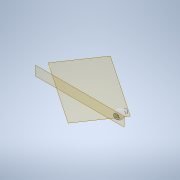
# Autodesk Inventor part: BallJoint
Saved by Autodesk Inventor 2020 (Build 240168000, 168)
## iProperties
Created: 2020-03-20
Part Number: BallJoint
Material: Generisch
Document SubType Name: Modeling
Designer: Fynn
Density: 1 g/cm^3
Appearance: Vorgabe
Author: Fynn
Autodesk Inventor part; units mm, degrees
ref_plane "YZ Plane" through (0, 0, 0) normal (1, 0, 0) x (0, 1, 0)
ref_plane "XZ Plane" through (0, 0, 0) normal (0, 1, 0) x (-1, 0, 0)
ref_plane "XY Plane" through (0, 0, 0) normal (0, 0, 1) x (1, 0, 0)
sketch "Skizze1" plane through (0, 0, 0) normal (0, 0, 1) x (1, 0, 0)
  circle A0 centre (75, -2.9684) radius 1.05 projected
  circle A1 centre (75, -2.9684) radius 2
  point P0 (0, 0)
  dimension "d0" = 4
  constraints: 1 centre point, 1 coincident
  measures "d0" diameter of A1
extrude "Extrusion1" add sketch "Skizze1" along normal blind 3
sketch "Skizze2" plane through (75, -2.9684, 3) normal (0, 0, 1) x (1, 0, 0)
  circle A0 centre (0, 0) radius 1.05 projected
  point P0 (-75, 2.9684)
ref_plane "Arbeitsebene2" through (75, -2.9684, 3) normal (-0.0001, 1, 0) x (-0.5613, -0.0001, 0.8276)
ref_plane "Arbeitsebene1" through (89.7752, 0.002, 14.6493) normal (-0.0001, 1, 0) x (-0.5613, -0.0001, 0.8276)
sketch "Skizze5" plane through (75, -2.9684, 3) normal (-0.0001, 1, 0) x (-0.5613, -0.0001, 0.8276)
  line L0 (1.1227, -1.6552) -> (-1.1227, 1.6552) projected
  line L1 (0, 0) -> (2.6411, 1.4229)
  circle A0 centre (2.6411, 1.4229) radius 4.25
  line L2 (2.6411, 1.4229) -> (6.3826, 3.4387)
  line L3 (1.1227, -1.6552) -> (-1.1227, 1.6552) projected
  line L4 (-1.3601, -3.3392) -> (-3.6054, -0.0288) projected
  line L5 (-1.6078, 1.3261) -> (-1.1227, 1.6552)
  line L6 (-3.6054, -0.0288) -> (-1.1227, 1.6552) projected
  point P0 (39.6166, -63.7532)
  point P1 (-0.9728, 1.669)
  point P2 (-1.1227, 1.6552)
  dimension "d6" = 3
  dimension "d8" = 8.5
  constraints: 6 end point, 2 collinear, 2 point on circle, 1 centre point, 1 coincident, 1 midpoint
  measures "d6" distance of L1.start L1.end
  measures "d8" diameter of A0
revolve "Umdrehung2" add sketch "Skizze5" angle 360 about axis through (74.6951, -2.9684, 5.9845) along (-0.1016, 0, 0.9948) picked at (0.1188, 2.1327) contours L0 L5 A0 L2 L1
extrude "Extrusion3" cut sketch "Skizze2" along normal through all
sketch "Skizze7" plane through (75, -2.9684, 3) normal (-0.0001, 1, 0) x (-0.5613, -0.0001, 0.8276)
  line L0 (-0.5894, 0.869) -> (5.2143, 4.8054) projected
  point P0 (39.6166, -63.7532)
ref_plane "Arbeitsebene4" through (76.05, -2.9682, 10.0127) normal (0, 0, 1) x (1, 0.0001, 0)
ref_plane "Arbeitsebene3" through (20.3611, -0.0073, 0) normal (0, 0, 1) x (1, 0.0001, 0)
sketch "Skizze8" plane through (76.05, -2.9682, 10.0127) normal (0, 0, 1) x (1, 0.0001, 0)
  line L0 (-1.05, 0) -> (0, -0.0001) projected
  circle A0 centre (-1.05, 0) radius 2.5
  point P0 (-76.0496, 2.9784)
  dimension "d12" = 5
  constraints: 1 centre point
  measures "d12" diameter of A0
extrude "Extrusion4" cut sketch "Skizze8" along normal mid plane 8
